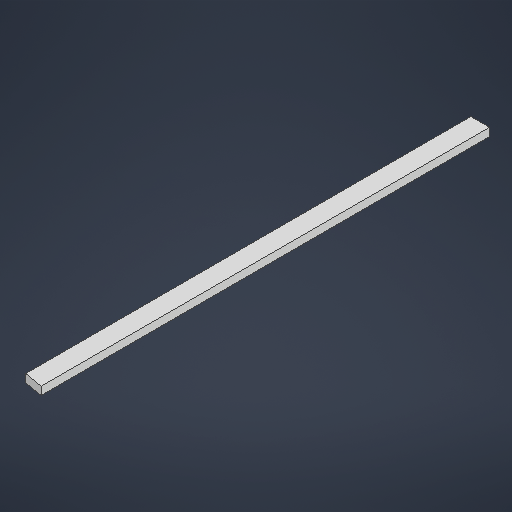
# Autodesk Inventor part: S_2x4x96b
Saved by Autodesk Inventor 2027.1 (Build 311270010, 270A)
## iProperties
Created: 2026-09-01
Part Number: S_2x4x96b
Material: Generic
Document SubType Name: Modeling
Designer: jorda
Density: 1 g/cm^3
Appearance: Default
Author: jorda
Autodesk Inventor part; units mm, degrees
ref_plane "YZ Plane" through (0, 0, 0) normal (1, 0, 0) x (0, 1, 0)
ref_plane "XZ Plane" through (0, 0, 0) normal (0, 1, 0) x (-1, 0, 0)
ref_plane "XY Plane" through (0, 0, 0) normal (0, 0, 1) x (1, 0, 0)
sketch "Sketch1" plane through (0, 0, 0) normal (0, 1, 0) x (-1, 0, 0)
  line L0 (0, -2133.6) -> (0, 0)
  line L1 (0, 0) -> (88.9, -15.6755)
  line L2 (0, 0) -> (116.206, 0) construction
  line L3 (88.9, -15.6755) -> (88.9, -2133.6)
  line L4 (0, 0) -> (0, -2133.6)
  line L5 (0, -2133.6) -> (88.9, -2133.6)
  dimension "d6" = 2133.6
  constraints: 12 end point, 1 horizontal, 1 parallel, 1 perpendicular
  measures "d6" distance of L0.start L0.end
extrude "Extrusion1" add sketch "Sketch1" along normal blind 38.1
body "Solid1"
